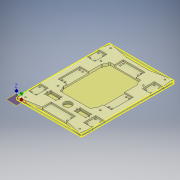
# Autodesk Inventor part: 3枚目
Saved by Autodesk Inventor 2018 (Build 220112000, 112)
## iProperties
Created: 2018-08-16
Part Number: 3枚目
Material: 一般
Document SubType Name: Modeling
Designer: shun2
Density: 1 g/cm^3
Appearance: 既定
Author: shun2
Autodesk Inventor part; units mm, degrees
ref_plane "YZ Plane" through (0, 0, 0) normal (1, 0, 0) x (0, 1, 0)
ref_plane "XZ Plane" through (0, 0, 0) normal (0, 1, 0) x (-1, 0, 0)
ref_plane "XY Plane" through (0, 0, 0) normal (0, 0, 1) x (1, 0, 0)
ref_plane "作業平面1" through (0, 0, 5.5) normal (0, 0, 1) x (1, 0, 0)
sketch "スケッチ3" plane through (0, 0, 5.5) normal (0, 0, 1) x (1, 0, 0)
  line L0 (0, 171.723921) -> (0, 23)
  line L1 (0, 23) -> (3, 0)
  line L2 (136, 23) -> (136, 171.723921)
  line L3 (136, 171.723921) -> (133.007871, 194.66358)
  line L4 (0, 23) -> (0, 75)
  line L5 (0, 127.723921) -> (0, 171.723921)
  line L6 (136, 171.723921) -> (136, 119.723921)
  line L7 (136, 67) -> (136, 23)
  circle A0 centre (11, 186.723921) radius 1.6
  circle A1 centre (125, 186.723921) radius 1.6
  circle A2 centre (11, 8) radius 1.6
  circle A3 centre (125, 8) radius 1.6
  line L8 (6.4, 186.723921) -> (15.6, 186.723921)
  line L9 (11, 182.123921) -> (11, 191.323921)
  line L10 (120.4, 186.723921) -> (129.6, 186.723921)
  line L11 (125, 182.123921) -> (125, 191.323921)
  line L12 (6.4, 8) -> (15.6, 8)
  line L13 (11, 3.4) -> (11, 12.6)
  line L14 (120.4, 8) -> (129.6, 8)
  line L15 (0, 127.723921) -> (0, 171.723921)
  line L16 (136, 171.723921) -> (136, 119.723921)
  line L17 (136, 67) -> (136, 23)
  line L18 (0, 23) -> (0, 75)
  line L19 (133, 0) -> (136, 23)
  line L20 (136, 46) -> (136, 23)
  line L21 (136, 23) -> (117.7, 23)
  line L22 (117.7, 23) -> (117.7, 48.5)
  line L23 (117.7, 48.5) -> (136, 48.5)
  line L24 (136, 48.5) -> (136, 23)
  line L25 (0, 23) -> (18.3, 23)
  line L26 (18.3, 23) -> (18.3, 48.5)
  line L27 (18.3, 48.5) -> (0, 48.5)
  line L28 (0, 48.5) -> (0, 23)
  line L29 (136, 171.723921) -> (117.7, 171.723921)
  line L30 (117.7, 171.723921) -> (117.7, 146.223921)
  line L31 (117.7, 146.223921) -> (136, 146.223921)
  line L32 (136, 146.223921) -> (136, 171.723921)
  line L33 (0, 171.723921) -> (18.3, 171.723921)
  line L34 (18.3, 171.723921) -> (18.3, 146.223921)
  line L35 (18.3, 146.223921) -> (0, 146.223921)
  line L36 (0, 146.223921) -> (0, 171.723921)
  circle A4 centre (132, 27) radius 1.6
  circle A5 centre (121.2, 27) radius 1.6
  circle A6 centre (132, 44.5) radius 1.6
  circle A7 centre (121.2, 44.5) radius 1.6
  circle A8 centre (132, 150.223921) radius 1.6
  circle A9 centre (132, 167.723921) radius 1.6
  circle A10 centre (121.2, 150.223921) radius 1.6
  circle A11 centre (121.2, 167.723921) radius 1.6
  circle A12 centre (14.8, 27) radius 1.6
  circle A13 centre (4, 27) radius 1.6
  circle A14 centre (14.8, 44.5) radius 1.6
  circle A15 centre (4, 44.5) radius 1.6
  circle A16 centre (14.8, 150.223921) radius 1.6
  circle A17 centre (4, 150.223921) radius 1.6
  circle A18 centre (14.8, 167.723921) radius 1.6
  circle A19 centre (4, 167.723921) radius 1.6
  line L37 (98, 8) -> (133, 0)
  line L38 (46.166731, 8) -> (3, 0)
  line L39 (98, 8) -> (46.166731, 8)
  line L40 (46.166731, 8) -> (46.166731, 26.3)
  line L41 (46.166731, 26.3) -> (98, 26.3)
  line L42 (98, 26.3) -> (98, 8)
  circle A20 centre (94, 12.65) radius 1.6
  circle A21 centre (94, 21.65) radius 1.6
  line L43 (68, 178.884921) -> (90.813, 178.884921)
  line L44 (90.813, 178.884921) -> (90.813, 160.584921)
  line L45 (90.813, 160.584921) -> (68, 160.584921)
  line L46 (133.007871, 194.66358) -> (90.813, 186.723921)
  line L47 (0, 171.723921) -> (2.992129, 194.66358)
  line L48 (68, 178.884921) -> (45.187, 178.884921)
  line L49 (45.187, 178.884921) -> (45.187, 160.584921)
  line L50 (45.187, 160.584921) -> (68, 160.584921)
  line L51 (2.992129, 194.66358) -> (45.187, 186.723921)
  circle A22 centre (86.313, 174.884921) radius 1.6
  circle A23 centre (86.313, 168.884921) radius 1.6
  line L52 (45.187, 186.723921) -> (90.813, 186.723921)
  circle A24 centre (49.687, 174.884921) radius 1.6
  circle A25 centre (49.687, 168.884921) radius 1.6
  line L53 (90.813, 160.584921) -> (45.187, 160.584921)
  line L54 (45.187, 160.584921) -> (45.187, 178.884921)
  line L55 (45.187, 178.884921) -> (90.813, 178.884921)
  line L56 (90.813, 178.884921) -> (90.813, 160.584921)
  point P0 (0, 0)
  point P1 (0, 179.723921)
  dimension "d134" = 18.3
  dimension "d137" = 3.2
  dimension "d139" = 3.2
  dimension "d196" = 22.813
  dimension "d197" = 18.3
  dimension "d198" = 3.2
  dimension "d199" = 4.5
  dimension "d200" = 4
  dimension "d202" = 3.2
  dimension "d203" = 10
  dimension "d256" = 26.139
  constraints: 114 end point, 26 centre point, 12 parallel, 9 horizontal, 7 perpendicular, 2 point on line
  measures "d134" distance of L39.end L40.end
  measures "d137" diameter of A20
  measures "d139" diameter of A21
  measures "d196" distance of L43.start L43.end
  measures "d197" distance of L43.end L44.end
  measures "d198" diameter of A22
  measures "d199" distance from line of A22.centre L44
  measures "d200" distance from line of L43 A22.centre
  measures "d202" diameter of A23
  measures "d203" distance from line of L43 A23.centre
  measures "d256" distance between parallel lines of L50 L52
ref_plane "作業平面6" through (0, 0, 5.5) normal (0, 0, 1) x (1, 0, 0)
ref_plane "作業平面7" through (0, 0, 5.5) normal (0, 0, -1) x (-1, 0, 0)
sketch "スケッチ9" plane through (0, 0, 5.5) normal (0, 0, -1) x (-1, 0, 0)
  line L0 (0, 146.223921) -> (0, 48.5)
  line L1 (0, 48.5) -> (0, 75)
  line L2 (0, 127.723921) -> (0, 146.223921)
  line L3 (0, 127.723921) -> (0, 146.223921)
  line L4 (0, 48.5) -> (0, 75)
  line L5 (-136, 171.723921) -> (-133.007871, 194.66358)
  circle A0 centre (-11, 186.723921) radius 1.6
  circle A1 centre (-125, 186.723921) radius 1.6
  circle A2 centre (-11, 8) radius 1.6
  circle A3 centre (-125, 8) radius 1.6
  line L6 (-6.4, 186.723921) -> (-15.6, 186.723921)
  line L7 (-11, 182.123921) -> (-11, 191.323921)
  line L8 (-120.4, 186.723921) -> (-129.6, 186.723921)
  line L9 (-125, 182.123921) -> (-125, 191.323921)
  line L10 (-6.4, 8) -> (-15.6, 8)
  line L11 (-11, 3.4) -> (-11, 12.6)
  line L12 (-120.4, 8) -> (-129.6, 8)
  line L13 (-133, 0) -> (-136, 23)
  line L14 (-136, 23) -> (-117.7, 23)
  line L15 (-117.7, 23) -> (-117.7, 48.5)
  line L16 (-117.7, 48.5) -> (-136, 48.5)
  line L17 (0, 23) -> (-18.3, 23)
  line L18 (-18.3, 23) -> (-18.3, 48.5)
  line L19 (-18.3, 48.5) -> (0, 48.5)
  line L20 (-117.7, 171.723921) -> (-117.7, 146.223921)
  line L21 (-117.7, 146.223921) -> (-136, 146.223921)
  circle A4 centre (-132, 27) radius 1.6
  circle A5 centre (-121.2, 27) radius 1.6
  circle A6 centre (-132, 44.5) radius 1.6
  circle A7 centre (-121.2, 44.5) radius 1.6
  circle A8 centre (-132, 150.223921) radius 1.6
  circle A9 centre (-132, 167.723921) radius 1.6
  circle A10 centre (-121.2, 150.223921) radius 1.6
  circle A11 centre (-121.2, 167.723921) radius 1.6
  circle A12 centre (-14.8, 27) radius 1.6
  circle A13 centre (-4, 27) radius 1.6
  circle A14 centre (-14.8, 44.5) radius 1.6
  circle A15 centre (-4, 44.5) radius 1.6
  line L22 (-98, 8) -> (-133, 0)
  line L23 (-46.166731, 8) -> (-3, 0)
  line L24 (-46.166731, 26.3) -> (-98, 26.3)
  line L25 (-98, 26.3) -> (-98, 8)
  circle A16 centre (-94, 12.65) radius 1.6
  circle A17 centre (-94, 21.65) radius 1.6
  circle A18 centre (-4, 150.223921) radius 1.6
  circle A19 centre (-14.8, 150.223921) radius 1.6
  circle A20 centre (-4, 167.723921) radius 1.6
  circle A21 centre (-14.8, 167.723921) radius 1.6
  line L26 (0, 0) -> (0, 23) construction
  line L27 (-136, 171.723921) -> (-117.7, 171.723921)
  line L28 (-117.7, 171.723921) -> (-136, 171.723921)
  line L29 (0, 48.5) -> (0, 146.223921) construction
  line L30 (0, 171.723921) -> (0, 236.188565) construction
  line L31 (0, 171.723921) -> (-3, 194.723921)
  line L32 (-18.3, 146.223921) -> (0, 146.223921)
  line L33 (-18.3, 171.723921) -> (-18.3, 146.223921)
  line L34 (-18.3, 146.223921) -> (0, 146.223921)
  line L35 (-18.3, 171.723921) -> (0, 171.723921)
  line L36 (0, 171.723921) -> (-18.3, 171.723921)
  line L37 (-136, 48.5) -> (-136, 146.223921)
  line L38 (-46.166731, 8) -> (-46.166731, 26.3)
  line L39 (0, 23) -> (-18.3, 23)
  line L40 (-3, 0) -> (0, 23)
  line L41 (-133.007871, 194.66358) -> (-90.813, 186.723921)
  line L42 (-136, 171.723921) -> (-133.007871, 194.66358)
  line L43 (-68, 178.884921) -> (-90.813, 178.884921)
  line L44 (-90.813, 178.884921) -> (-90.813, 160.584921)
  circle A22 centre (-86.313, 175.719753) radius 1.6
  circle A23 centre (-86.313, 169.719753) radius 1.6
  line L45 (-90.813, 160.584921) -> (-68, 160.584921)
  line L46 (-45.187, 160.584921) -> (-68, 160.584921)
  line L47 (-45.187, 178.884921) -> (-45.187, 160.584921)
  circle A24 centre (-48.579797, 169.719753) radius 1.6
  circle A25 centre (-48.579797, 175.719753) radius 1.6
  line L48 (-68, 178.884921) -> (-45.187, 178.884921)
  line L49 (-2.992129, 194.66358) -> (-45.187, 186.723921)
  line L50 (0, 171.723921) -> (-2.992129, 194.66358)
  line L51 (-45.187, 186.723921) -> (-90.813, 186.723921)
  point P0 (0, 179.723921)
  point P1 (-90.166731, 179.719753)
  point P2 (-42, 173.073921)
  point P3 (-42, 182.073921)
  dimension "d150" = 3.2
  dimension "d151" = 3.2
  dimension "d152" = 3.2
  dimension "d153" = 3.2
  dimension "d257" = 26.139
  constraints: 88 end point, 26 centre point, 5 vertical, 2 horizontal, 1 collinear, 1 perpendicular, 1 point on line, 4 other
  measures "d150" diameter of A18
  measures "d151" diameter of A19
  measures "d152" diameter of A20
  measures "d153" diameter of A21
  measures "d257" distance between parallel lines of L45 L51
extrude "押し出し9" add sketch "スケッチ9" against normal blind 5.5 contours L0 L19 L18 L17 L40 L23 L38 L24 L25 L22 L13 L14 L15 L16 L37 L21 L20 L27 L5 L41 L51 L49 L31 L35 L33 L32
ref_plane "作業平面8" through (0, 0, 5.5) normal (0, 0, -1) x (-1, 0, 0)
sketch "スケッチ10" plane through (0, 0, 5.5) normal (0, 0, -1) x (-1, 0, 0)
  line L0 (0, 0) -> (0, 225.606383) construction
  circle A0 centre (-68, 39.746288) radius 8
  circle A1 centre (-112.199225, 40.36196) radius 1.15
  line L1 (-87.699225, 46.36196) -> (-110.699225, 46.36196)
  line L2 (-110.699225, 46.36196) -> (-110.699225, 34.36196)
  circle A2 centre (-86.199225, 40.36196) radius 1.15
  line L3 (-110.699225, 34.36196) -> (-87.699225, 34.36196)
  line L4 (-87.699225, 34.36196) -> (-87.699225, 46.36196)
  circle A3 centre (-49.800775, 40.36196) radius 1.15
  line L5 (-48.300775, 34.36196) -> (-48.300775, 46.36196)
  line L6 (-48.300775, 46.36196) -> (-25.300775, 46.36196)
  line L7 (-25.300775, 34.36196) -> (-48.300775, 34.36196)
  line L8 (-25.300775, 46.36196) -> (-25.300775, 34.36196)
  circle A4 centre (-23.800775, 40.36196) radius 1.15
  constraints: 18 end point, 5 centre point, 1 vertical
extrude "押し出し10" cut sketch "スケッチ10" against normal blind 5.5
sketch "スケッチ13" plane through (0, 0, 11) normal (0, 0, 1) x (1, 0, 0)
  line L0 (105.679, 75.617464) -> (105.679, 121.243464)
  line L1 (105.679, 75.617464) -> (123.979613, 75.617464)
  line L2 (123.979613, 121.243464) -> (123.979613, 75.617464)
  line L3 (105.679, 121.243464) -> (123.979613, 121.243464)
  line L4 (136, 48.5) -> (136, 146.223921)
  line L5 (30.321, 75.617464) -> (30.321, 121.243464)
  line L6 (30.321, 75.617464) -> (12.020387, 75.617464)
  line L7 (12.020387, 121.243464) -> (12.020387, 75.617464)
  line L8 (30.321, 121.243464) -> (12.020387, 121.243464)
  point P0 (105.962537, 75.617464)
  point P1 (244.119648, 130.817382)
  point P2 (0, 62.936013)
  point P3 (121.359387, 75.617464)
  point P4 (123.979, 75.617464)
  point P5 (30.037463, 75.617464)
  point P6 (14.640613, 75.617464)
  point P7 (12.021, 75.617464)
  dimension "d207" = 45.626
  dimension "d226" = 30.321
  constraints: 16 end point, 2 point on line
  measures "d207" distance between parallel lines of L3 L1
  measures "d226" distance between parallel lines of L0 L4
extrude "押し出し13" cut sketch "スケッチ13" against normal blind 2.5
sketch "スケッチ14" plane through (132, 67.436013, 11) normal (0, 0, 1) x (1, 0, 0)
  circle A0 centre (-18.020387, 49.307451) radius 1.6
  circle A1 centre (-12.020387, 49.307451) radius 1.6
  circle A2 centre (-18.020387, 12.681451) radius 1.6
  circle A3 centre (-12.020387, 12.681451) radius 1.6
  circle A4 centre (-6, 0) radius 1.642331
  circle A5 centre (-109.979613, 49.307451) radius 1.6
  circle A6 centre (-115.979613, 49.307451) radius 1.6
  circle A7 centre (-109.979613, 12.681451) radius 1.6
  circle A8 centre (-115.979613, 12.681451) radius 1.6
  circle A9 centre (-115.979613, 49.307451) radius 1.6
  circle A10 centre (-109.979613, 49.307451) radius 1.6
  circle A11 centre (-115.979613, 12.681451) radius 1.6
  circle A12 centre (-109.979613, 12.681451) radius 1.6
  point P0 (-132.5, -84.334225)
  dimension "d252" = 3.2
  dimension "d253" = 3.2
  dimension "d254" = 3.2
  dimension "d255" = 3.2
  constraints: 12 centre point, 4 coincident
  measures "d252" diameter of A9
  measures "d253" diameter of A10
  measures "d254" diameter of A11
  measures "d255" diameter of A12
extrude "押し出し14" cut sketch "スケッチ14" against normal blind 5.5 contours A0 | A1 | A2 | A3 | A5 | A6 | A7 | A8
extrude "押し出し15" add sketch "スケッチ3" along normal blind 2.5 contours L33 L34 L35 L0 | L27 L26 L25 L0 | L2 L31 L30 L29 | L40 L41 L42 L39 | L2 L21 L22 L23 | L43 L44 L45 L50 L49 L48
sketch "スケッチ15" plane through (0, 0, 5.5) normal (0, 0, -1) x (-1, 0, 0)
  arc A0 (-25.727023, 62.993307) -> (-22.501223, 62.993307) centre (-24.114123, 62.993307) ccw
  arc A1 (-22.501223, 62.993307) -> (-25.727023, 62.993307) centre (-24.114123, 62.993307) ccw
  arc A2 (-25.727023, 62.993307) -> (-22.501223, 62.993307) centre (-24.114123, 62.993307) ccw
  arc A3 (-22.501223, 62.993307) -> (-25.727023, 62.993307) centre (-24.114123, 62.993307) ccw
  arc A4 (-25.727023, 153.163307) -> (-22.501223, 153.163307) centre (-24.114123, 153.163307) ccw
  arc A5 (-22.501223, 153.163307) -> (-25.727023, 153.163307) centre (-24.114123, 153.163307) ccw
  arc A6 (-25.727023, 153.163307) -> (-22.501223, 153.163307) centre (-24.114123, 153.163307) ccw
  arc A7 (-22.501223, 153.163307) -> (-25.727023, 153.163307) centre (-24.114123, 153.163307) ccw
  arc A8 (-114.627023, 153.163307) -> (-111.401223, 153.163307) centre (-113.014123, 153.163307) ccw
  arc A9 (-111.401223, 153.163307) -> (-114.627023, 153.163307) centre (-113.014123, 153.163307) ccw
  arc A10 (-114.627023, 153.163307) -> (-111.401223, 153.163307) centre (-113.014123, 153.163307) ccw
  arc A11 (-111.401223, 153.163307) -> (-114.627023, 153.163307) centre (-113.014123, 153.163307) ccw
  arc A12 (-114.627023, 62.993307) -> (-111.401223, 62.993307) centre (-113.014123, 62.993307) ccw
  arc A13 (-111.401223, 62.993307) -> (-114.627023, 62.993307) centre (-113.014123, 62.993307) ccw
  arc A14 (-114.627023, 62.993307) -> (-111.401223, 62.993307) centre (-113.014123, 62.993307) ccw
  arc A15 (-111.401223, 62.993307) -> (-114.627023, 62.993307) centre (-113.014123, 62.993307) ccw
  circle A16 centre (-113.014123, 153.163307) radius 1.6
  line L0 (-117.7, 146.223921) -> (-117.7, 171.723921)
  line L1 (-100.7, 160.585295) -> (-35.3, 160.585295)
  line L2 (-35.3, 55.585295) -> (-100.7, 55.585295)
  arc A17 (-105.679185, 148.56448) -> (-100.7, 160.585295) centre (-117.7, 160.585295) ccw
  arc A18 (-100.7, 55.585295) -> (-105.679185, 67.60611) centre (-117.7, 55.585295) ccw
  arc A19 (-30.320815, 67.60611) -> (-35.3, 55.585295) centre (-18.3, 55.585295) ccw
  line L3 (-136, 171.723921) -> (-136, 23)
  line L4 (-105.679185, 67.60611) -> (-105.679185, 148.56448)
  line L5 (-30.320815, 67.60611) -> (-30.320815, 148.183615)
  arc A20 (-35.3, 160.585295) -> (-30.725766, 148.983556) centre (-18.3, 160.585295) ccw
  arc A21 (-35.3, 160.585295) -> (-30.320815, 148.56448) centre (-18.3, 160.585295) ccw
  line L6 (-30.320815, 148.183615) -> (-30.320815, 148.56448)
  circle A22 centre (-24.114123, 62.993307) radius 1.6
  circle A23 centre (-24.114123, 153.163307) radius 1.6
  circle A24 centre (-113.014123, 153.163307) radius 1.6
  circle A25 centre (-113.014123, 62.993307) radius 1.6
  point P0 (0, 0)
  point P1 (-119.147223, 157.649707)
  point P2 (-136, 146.223921)
  point P3 (-136, 48.5)
  dimension "d233" = 34
  dimension "d235" = 34
  dimension "d236" = 34
  dimension "d238" = 3.2
  dimension "d239" = 3.2
  dimension "d240" = 3.2
  dimension "d241" = 3.2
  constraints: 42 point on circle, 25 centre point, 10 end point, 5 coincident, 2 parallel, 2 vertical, 1 concentric, 1 horizontal
  measures "d233" diameter of A17
  measures "d235" diameter of A18
  measures "d236" diameter of A19
  measures "d238" diameter of A22
  measures "d239" diameter of A23
  measures "d240" diameter of A24
  measures "d241" diameter of A25
sketch "スケッチ15 outline for 押し出し16" plane through (0, 0, 5.5) normal (0, 0, -1) x (-1, 0, 0)
  circle A0 centre (-113.014123, 153.163307) radius 1.6
  circle A1 centre (-24.114123, 62.993307) radius 1.6
  circle A2 centre (-24.114123, 153.163307) radius 1.6
  circle A3 centre (-113.014123, 62.993307) radius 1.6
  line L0 (-30.320815, 67.60611) -> (-30.320815, 148.56448)
  arc A4 (-35.3, 160.585295) -> (-30.320815, 148.56448) centre (-18.3, 160.585295) ccw
  line L1 (-100.7, 160.585295) -> (-35.3, 160.585295)
  arc A5 (-105.679185, 148.56448) -> (-100.7, 160.585295) centre (-117.7, 160.585295) ccw
  line L2 (-105.679185, 67.60611) -> (-105.679185, 148.56448)
  arc A6 (-100.7, 55.585295) -> (-105.679185, 67.60611) centre (-117.7, 55.585295) ccw
  line L3 (-35.3, 55.585295) -> (-100.7, 55.585295)
  arc A7 (-30.320815, 67.60611) -> (-35.3, 55.585295) centre (-18.3, 55.585295) ccw
extrude "押し出し16" cut sketch "スケッチ15 outline for 押し出し16" against normal blind 5.5
fillet "フィレット1" radius 2 8 edges at (105.6792, 148.5645, 8.25) (105.6792, 67.6061, 8.25) (100.7, 55.5853, 8.25) (100.7, 160.5853, 8.25) (35.3, 160.5853, 8.25) (30.3208, 148.5645, 8.25) (30.3208, 67.6061, 8.25) (35.3, 55.5853, 8.25)
sketch "スケッチ16" plane through (0, 0, 11) normal (0, 0, 1) x (1, 0, 0)
  line L0 (25.300775, 34.36196) -> (25.300775, 46.36196)
  circle A0 centre (25.300775, 34.36196) radius 1
  circle A1 centre (25.300775, 46.36196) radius 1
  line L1 (25.300775, 46.36196) -> (48.300775, 46.36196)
  circle A2 centre (48.300775, 46.36196) radius 1
  circle A3 centre (48.300775, 34.36196) radius 1
  line L2 (110.699225, 34.36196) -> (87.699225, 34.36196)
  circle A4 centre (87.699225, 34.36196) radius 1
  circle A5 centre (87.699225, 46.36196) radius 1
  line L3 (110.699225, 46.36196) -> (110.699225, 34.36196)
  circle A6 centre (110.699225, 46.36196) radius 1
  circle A7 centre (110.699225, 34.36196) radius 1
  point P0 (0, 0)
  dimension "d259" = 2
  dimension "d260" = 2
  dimension "d261" = 2
  dimension "d262" = 2
  dimension "d263" = 2
  dimension "d264" = 2
  dimension "d265" = 2
  dimension "d266" = 2
  constraints: 8 centre point, 2 coincident
  measures "d259" diameter of A0
  measures "d260" diameter of A1
  measures "d261" diameter of A2
  measures "d262" diameter of A3
  measures "d263" diameter of A4
  measures "d264" diameter of A5
  measures "d265" diameter of A6
  measures "d266" diameter of A7
extrude "押し出し17" cut sketch "スケッチ16" against normal blind 10
